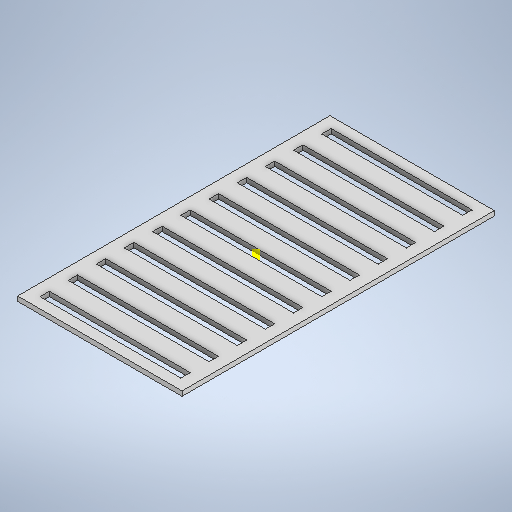
# Autodesk Inventor part: Part3
Saved by Autodesk Inventor 2025 (Build 290162000, 162)
## iProperties
Created: 2024-06-18
Part Number: Part3
Material: Generic
Document SubType Name: Modeling
Designer: Isaac
Density: 1 g/cm^3
Appearance: Default
Author: Isaac
Autodesk Inventor part; units mm, degrees
ref_plane "YZ Plane" through (0, 0, 0) normal (1, 0, 0) x (0, 1, 0)
ref_plane "XZ Plane" through (0, 0, 0) normal (0, 1, 0) x (-1, 0, 0)
ref_plane "XY Plane" through (0, 0, 0) normal (0, 0, 1) x (1, 0, 0)
sketch "Sketch1" plane through (0, 0, 0) normal (0, 0, 1) x (1, 0, 0)
  point P0 (0, 0)
sketch "Sketch2" plane through (0, 0, 0) normal (0, 1, 0) x (-1, 0, 0)
  line L0 (350, 665) -> (-350, 665)
  line L1 (-350, 665) -> (-350, -665)
  line L2 (-350, -665) -> (350, -665)
  line L3 (350, -665) -> (350, 665)
  line L4 (350, 665) -> (-350, -665) construction
  line L5 (-350, 665) -> (350, -665) construction
  point P0 (0, 0)
  dimension "d0" = 700
  dimension "d1" = 1330
  constraints: 12 end point, 2 midpoint, 2 parallel, 1 horizontal, 1 perpendicular
  measures "d0" distance of L0.start L0.end
  measures "d1" distance of L2.end L0.start
extrude "Extrusion1" add sketch "Sketch2" along normal blind 20
sketch "Sketch3" plane through (0, 20, 0) normal (0, 1, 0) x (1, 0, 0)
  line L0 (-300, -20) -> (300, -20)
  line L1 (300, -20) -> (300, 20)
  line L2 (300, 20) -> (-300, 20)
  line L3 (-300, 20) -> (-300, -20)
  line L4 (-300, -20) -> (300, 20) construction
  line L5 (300, -20) -> (-300, 20) construction
  point P0 (0, 0)
  point P1 (0, 0)
  dimension "d4" = 40
  dimension "d5" = 600
  constraints: 12 end point, 2 midpoint, 2 parallel, 1 coincident, 1 horizontal, 1 perpendicular
  measures "d4" distance of L2.end L0.start
  measures "d5" distance of L0.start L0.end
extrude "Extrusion2" cut sketch "Sketch3" against normal through all
sketch "Sketch4" plane through (0, 20, 0) normal (0, 1, 0) x (1, 0, 0)
  line L0 (-300, -140) -> (300, -140)
  line L1 (300, -140) -> (300, -100)
  line L2 (300, -100) -> (-300, -100)
  line L3 (-300, -100) -> (-300, -140)
  line L4 (-300, -140) -> (300, -100) construction
  line L5 (300, -140) -> (-300, -100) construction
  line L6 (-300, 100) -> (300, 100)
  line L7 (300, 100) -> (300, 140)
  line L8 (300, 140) -> (-300, 140)
  line L9 (-300, 140) -> (-300, 100)
  line L10 (-300, 100) -> (300, 140) construction
  line L11 (300, 100) -> (-300, 140) construction
  point P0 (0, 0)
  point P1 (0, -120)
  point P2 (0, 120)
  dimension "d8" = 0
  dimension "d9" = 120
  dimension "d10" = 600
  dimension "d11" = 40
  dimension "d12" = 120
  dimension "d13" = 40
  constraints: 24 end point, 4 midpoint, 4 parallel, 2 horizontal, 2 perpendicular
  measures "d8" horizontal distance of point (0, 0) point (0, -120)
  measures "d9" distance of point (0, 0) point (0, -120)
  measures "d10" distance of L0.start L0.end
  measures "d11" distance of L0.end L1.end
  measures "d12" distance of point (0, 120) point (0, 0)
  measures "d13" distance of L8.end L6.start
extrude "Extrusion3" cut sketch "Sketch4" against normal through all
sketch "Sketch5" plane through (0, 20, 0) normal (0, 1, 0) x (1, 0, 0)
  line L0 (-300, -260) -> (300, -260)
  line L1 (300, -260) -> (300, -220)
  line L2 (300, -220) -> (-300, -220)
  line L3 (-300, -220) -> (-300, -260)
  line L4 (-300, -260) -> (300, -220) construction
  line L5 (300, -260) -> (-300, -220) construction
  line L6 (-300, 220) -> (300, 220)
  line L7 (300, 220) -> (300, 260)
  line L8 (300, 260) -> (-300, 260)
  line L9 (-300, 260) -> (-300, 220)
  line L10 (-300, 220) -> (300, 260) construction
  line L11 (300, 220) -> (-300, 260) construction
  line L12 (-300, -380) -> (300, -380)
  line L13 (300, -380) -> (300, -340)
  line L14 (300, -340) -> (-300, -340)
  line L15 (-300, -340) -> (-300, -380)
  line L16 (-300, -380) -> (300, -340) construction
  line L17 (300, -380) -> (-300, -340) construction
  line L18 (-300, 340) -> (300, 340)
  line L19 (300, 340) -> (300, 380)
  line L20 (300, 380) -> (-300, 380)
  line L21 (-300, 380) -> (-300, 340)
  line L22 (-300, 340) -> (300, 380) construction
  line L23 (300, 340) -> (-300, 380) construction
  line L24 (-300, -460) -> (300, -460)
  line L25 (300, -460) -> (300, -500)
  line L26 (300, -500) -> (-300, -500)
  line L27 (-300, -500) -> (-300, -460)
  line L28 (-300, -460) -> (300, -500) construction
  line L29 (300, -460) -> (-300, -500) construction
  line L30 (300, 500) -> (-300, 500)
  line L31 (-300, 500) -> (-300, 460)
  line L32 (-300, 460) -> (300, 460)
  line L33 (300, 460) -> (300, 500)
  line L34 (300, 500) -> (-300, 460) construction
  line L35 (-300, 500) -> (300, 460) construction
  line L36 (-300, 620) -> (300, 620)
  line L37 (300, 620) -> (300, 580)
  line L38 (300, 580) -> (-300, 580)
  line L39 (-300, 580) -> (-300, 620)
  line L40 (-300, 620) -> (300, 580) construction
  line L41 (300, 620) -> (-300, 580) construction
  line L42 (-300, -580) -> (300, -580)
  line L43 (300, -580) -> (300, -620)
  line L44 (300, -620) -> (-300, -620)
  line L45 (-300, -620) -> (-300, -580)
  line L46 (-300, -580) -> (300, -620) construction
  line L47 (300, -580) -> (-300, -620) construction
  point P0 (0, 0)
  point P1 (0, -240)
  point P2 (0, 240)
  point P3 (0, -360)
  point P4 (0, 360)
  point P5 (0, -480)
  point P6 (0, 480)
  point P7 (0, 600)
  point P8 (0, -600)
  dimension "d16" = 600
  dimension "d17" = 600
  dimension "d18" = 0
  dimension "d19" = 240
  dimension "d20" = 40
  dimension "d21" = 40
  dimension "d22" = 120
  dimension "d23" = 600
  dimension "d24" = 240
  dimension "d25" = 40
  dimension "d26" = 120
  dimension "d27" = 40
  dimension "d28" = 120
  dimension "d29" = 40
  dimension "d30" = 600
  dimension "d31" = 40
  dimension "d32" = 600
  dimension "d33" = 0
  dimension "d34" = 120
  dimension "d35" = 600
  dimension "d36" = 0
  dimension "d37" = 40
  dimension "d38" = 120
  dimension "d39" = 40
  dimension "d40" = 120
  constraints: 96 end point, 16 midpoint, 16 parallel, 8 horizontal, 8 perpendicular, 2 point on line
  measures "d16" distance of L0.start L0.end
  measures "d17" distance of L19.end L20.end
  measures "d18" horizontal distance of point (0, 240) point (0, 360)
  measures "d19" distance of point (0, -240) point (0, 0)
  measures "d20" distance between parallel lines of L2 L0
  measures "d21" distance of L14.end L12.start
  measures "d22" distance of point (0, -240) point (0, -360)
  measures "d23" distance of L12.start L12.end
  measures "d24" distance of point (0, 0) point (0, 240)
  measures "d25" distance of L6.end L7.end
  measures "d26" distance of point (0, 240) point (0, 360)
  measures "d27" distance of L18.end L19.end
  measures "d28" distance of point (0, -360) point (0, -480)
  measures "d29" distance of L24.end L25.end
  measures "d30" distance of L25.end L26.end
  measures "d31" distance between parallel lines of L30 L32
  measures "d32" distance of L31.end L32.end
  measures "d33" horizontal distance of point (0, 360) point (0, 480)
  measures "d34" distance of point (0, 360) point (0, 480)
  measures "d35" distance of L36.start L36.end
  measures "d36" horizontal distance of point (0, 480) point (0, 600)
  measures "d37" distance of L36.end L37.end
  measures "d38" distance of point (0, 600) point (0, 480)
  measures "d39" distance of L42.end L43.end
  measures "d40" distance of point (0, -480) point (0, -600)
sketch "Sketch6" plane through (0, 20, 0) normal (0, 1, 0) x (1, 0, 0)
  point P0 (0, 0)
extrude "Extrusion4" cut sketch "Sketch5" against normal through all
body "Solid1"
